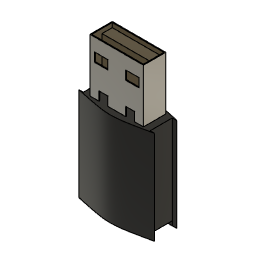
USBWIFI v2 v1 (Autodesk Fusion 360 design; units mm, degrees)
Autodesk Fusion 360 part; units mm, degrees
sketch "草图1" plane through (0, 0, 0) normal (0, 0, 1) x (1, 0, 0)
  line L0 (0, 0) -> (15, 0)
  line L1 (15, 0) -> (15, 5)
  line L2 (15, 5) -> (0, 5)
  line L3 (0, 5) -> (0, 0)
  spline S0 degree 2 poles (-1.0359, 5) (7.5, 6.9661) (16, 5) knots 0 0 0 1.728929 1.728929 1.728929 weights 1 3 1
  spline S1 degree 2 poles (-1, 0) (7.5, -1.8518) (16, 0) knots 0 0 0 1.722544 1.722544 1.722544 weights 1 3 1
  line L4 (16, 5) -> (15, 5)
  line L5 (-1.0359, 5) -> (0, 5)
  line L6 (-1, 0) -> (0, 0)
  line L7 (15, 0) -> (16, 0)
  dimension "d1" = 15
  dimension "d2" = 5
  constraint horizontal L0
  constraint vertical L1
  constraint horizontal L2
  constraint vertical L3
  constraint coincident L0.start L3.end
  constraint perpendicular L3 L5
  constraint perpendicular L3 L6
  constraint perpendicular L1 L7
  measures "d1" distance of L0.start L0.end
  measures "d2" distance of L0.start L2.end
extrude "拉伸1" add sketch "草图1" along normal blind 20 contours L0 L1 L2 L3
extrude "拉伸2" add sketch "草图1" along normal blind 20 and the other way blind 1 contours L0 S1 L6 L7 | L2 S0 L4 L5
sketch "草图2" plane through (0, 0, 20) normal (0, 0, 1) x (-1, 0, 0)
  line L0 (0, -5) -> (0, 0)
  line L1 (0, 0) -> (1, 0)
  spline S0 degree 2 poles (1, 0) (-7.5, 1.8518) (-16, 0) knots 0 0 0 1.722544 1.722544 1.722544 weights 1 3 1
  line L2 (-16, 0) -> (-15, 0)
  line L3 (-15, 0) -> (-15, -5)
  line L4 (-15, -5) -> (-16, -5)
  spline S1 degree 2 poles (-16, -5) (-7.5, -6.9661) (1.0359, -5) knots -1.728929 -1.728929 -1.728929 0 0 0 weights 1 3 1
  line L5 (1.0359, -5) -> (0, -5)
  line L6 (-1.5, -5.0039) -> (-13.5, -5.0039)
  line L7 (-13.5, -5.0039) -> (-13.5, -0.0039)
  line L8 (-13.5, -0.0039) -> (-1.5, -0.0039)
  line L9 (-1.5, -0.0039) -> (-1.5, -5.0039)
  line L10 (-13.3, -0.2039) -> (-1.7, -0.2039)
  line L11 (-1.7, -0.2039) -> (-1.7, -4.8039)
  line L12 (-1.7, -4.8039) -> (-13.3, -4.8039)
  line L13 (-13.3, -4.8039) -> (-13.3, -0.2039)
  line L14 (-1.7, -2.5039) -> (-13.3, -2.5039)
  dimension "d11" = 12
  dimension "d12" = 5
  dimension "d13" = 1.5
  dimension "d14" = 0.2
  constraint horizontal L6
  constraint vertical L7
  constraint horizontal L8
  constraint vertical L9
  constraint midpoint L11 L14.start
  constraint midpoint L13 L14.end
  measures "d11" distance of L6.start L6.end
  measures "d12" distance of L6.start L8.end
  measures "d13" distance of L0 L9
extrude "拉伸3" add sketch "草图2" along normal blind 12 contours L6 L7 L8 L9
extrude "拉伸4" add sketch "草图2" along normal blind 11 contours L11 L12 L13 L14
sketch "草图3" plane through (0, 0.0039, 0) normal (0, -1, 0) x (1, 0, 0)
  line L0 (1.5, 20) -> (13.5, 20)
  line L1 (13.5, 20) -> (13.5, 32)
  line L2 (13.5, 32) -> (1.5, 32)
  line L3 (1.5, 32) -> (1.5, 20)
  line L4 (7.5, 20) -> (7.5, 32) construction
  line L5 (3.5, 20) -> (5.5, 20)
  line L6 (5.5, 20) -> (5.5, 22)
  line L7 (5.5, 22) -> (3.5, 22)
  line L8 (3.5, 22) -> (3.5, 20)
  line L9 (2.5, 29.0815) -> (5.5, 29.0815)
  line L10 (5.5, 29.0815) -> (5.5, 27.0815)
  line L11 (5.5, 27.0815) -> (2.5, 27.0815)
  line L12 (2.5, 27.0815) -> (2.5, 29.0815)
  line L13 (12.5, 29.0815) -> (9.5, 29.0815)
  line L14 (12.5, 27.0815) -> (12.5, 29.0815)
  line L15 (9.5, 29.0815) -> (9.5, 27.0815)
  line L16 (9.5, 27.0815) -> (12.5, 27.0815)
  line L17 (9.5, 22) -> (11.5, 22)
  line L18 (11.5, 22) -> (11.5, 20)
  line L19 (9.5, 20) -> (9.5, 22)
  line L20 (11.5, 20) -> (9.5, 20)
  dimension "d19" = 2
  dimension "d20" = 2
  dimension "d21" = 2
  dimension "d22" = 3
  dimension "d23" = 2
  dimension "d24" = 2
  constraint midpoint L0 L4.start
  constraint midpoint L2 L4.end
  constraint horizontal L5
  constraint vertical L6
  constraint horizontal L7
  constraint vertical L8
  constraint coincident L0 L5.start
  constraint horizontal L9
  constraint vertical L10
  constraint horizontal L11
  constraint vertical L12
  constraint symmetric L4 L5.start L18.end
  constraint symmetric L4 L5.end L19.start
  constraint symmetric L4 L6.end L17.start
  constraint symmetric L4 L7.end L17.end
  constraint symmetric L4 L9.start L13.start
  constraint symmetric L4 L9.end L13.end
  constraint symmetric L4 L10.end L15.end
  constraint symmetric L4 L11.end L14.start
  measures "d19" distance of L5.start L5.end
  measures "d20" distance of L5.start L7.end
  measures "d21" distance of L4 L6
  measures "d22" distance of L9.start L9.end
  measures "d23" distance of L9.start L11.end
  measures "d24" distance of L4 L10
extrude "拉伸5" cut sketch "草图3" against normal up to surface (0.2 mm away) contours L0 L5 L6 L7 L8 | L0 L17 L18 L19 L20 | L9 L10 L11 L12 | L13 L14 L15 L16
